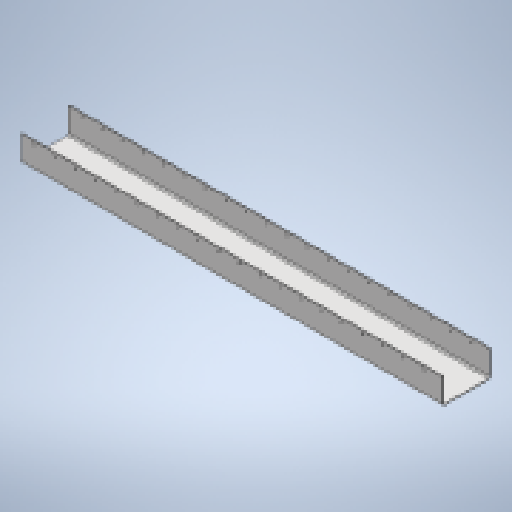
# Autodesk Inventor part: MSC 081 pillar 1_CPY
Saved by Autodesk Inventor 2025 (Build 290162010, 162A)
## iProperties
Created: 2024-06-25
Part Number: MSC 081 pillar 1_CPY
Material: Stainless Steel
Document SubType Name: Sheet Metal
Designer: admin
Density: 8 g/cm^3
Sheet Metal Rule: AISI304 3mm Die 32
Appearance: Default
Author: admin
Autodesk Inventor part; units mm, degrees
ref_plane "YZ Plane" through (0, 0, 0) normal (1, 0, 0) x (0, 1, 0)
ref_plane "XZ Plane" through (0, 0, 0) normal (0, 1, 0) x (-1, 0, 0)
ref_plane "XY Plane" through (0, 0, 0) normal (0, 0, 1) x (1, 0, 0)
sketch3d "3D Sketch1"
sketch "Sketch1" plane through (0, 0, 0) normal (0, 0, 1) x (1, 0, 0)
  line L0 (-650, 75) -> (650, 75)
  line L1 (650, 75) -> (650, -75)
  line L2 (650, -75) -> (-650, -75)
  line L3 (-650, -75) -> (-650, 75)
  line L4 (-650, 75) -> (650, -75) construction
  line L5 (650, 75) -> (-650, -75) construction
  point P0 (0, 0)
  dimension "d5" = 1300
  dimension "d30" = 150
  measures "d5" distance of L1.end L2.end
  measures "d30" distance of L2.end L0.start
extrude "Plate1" add sketch "Sketch1" along normal blind 3
sketch "Sketch6" plane through (650, -72, 0) normal (0, -1, 0) x (1, 0, 0)
  line L0 (-1300, 0) -> (0, 0)
  line L1 (0, 0) -> (0, 80)
  line L2 (0, 80) -> (-1300, 80)
  line L3 (-1300, 80) -> (-1300, 0)
  constraints: 6 end point, 1 horizontal, 1 perpendicular, 1 vertical
edge flange "Flange4" height 80 angle 90 thickness 3 bend radius 5 thickness toward (0, -1, 0) relief round relief width 3 relief depth 1.5 corner gap 5 corner form 0 edges at (0, -75, 3) (0, 75, 3) wall of the first edge with corners at (-650, -72, 0) (650, -72, 0) (650, -72, 80) (-650, -72, 80)
bend "Bend4"
corner "Corner4"
sketch "Sketch8" plane through (0, 0, 0) normal (0, 1, 0) x (-1, 0, 0)
  line L0 (650, 8) -> (-650, 8) construction
  line L1 (-650, 80) -> (-650, 8) construction
  line L2 (650, 80) -> (-650, 80) construction
  line L3 (650, 8) -> (650, 80) projected
  circle A0 centre (-594, 70) radius 2.5
  point P0 (0, 0)
  dimension "d73" = 5
  dimension "d74" = 10
  dimension "d75" = 56
  constraints: 1 centre point
  measures "d73" diameter of A0
  measures "d74" distance from line of L2 A0.centre
  measures "d75" distance from line of L1 A0.centre
extrude "Extrusion3" cut sketch "Sketch8" along normal through all both and the other way through all
pattern_linear "Rectangular Pattern1" count 22 spacing 63 along (-1, 0, 0) of "Extrusion3"
equation "\"d6\" = Thickness"
equation "\"d60\" = BendReliefWidth"
equation "\"d61\" = BendReliefDepth"
equation "\"d62\" = MinimumRemnant"
equation "\"d63\" = TransitionRadius"
equation "\"d66\" = BendRadius"
equation "\"d67\" = CornerReliefSize"
equation "\"d68\" = GapSize"
equation "\"d69\" = JacobiRadiusSize"
equation "\"BendReliefWidth\" = Thickness"
equation "\"BendReliefDepth\" = 0.5 * Thickness"
equation "\"CornerReliefSize\" = 4 * Thickness"
equation "\"MinimumRemnant\" = 2 * Thickness"
equation "\"TransitionRadius\" = BendRadius"
equation "\"JacobiRadiusSize\" = BendRadius"
equation "\"GapSize\" = Thickness"
equation "\"Thickness\" = 3"
equation "\"BendRadius\" = 5"
body "Solid1"
